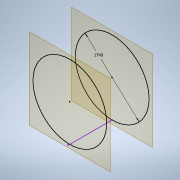
# Autodesk Inventor part: bok
Saved by Autodesk Inventor 2021 (Build 250183000, 183)
## iProperties
Created: 2021-09-19
Part Number: bok
Material: Ogólny
Document SubType Name: Konstrukcja blachowa
Designer: wojwo
Density: 1 g/cm^3
Sheet Metal Rule: Domyślny
Appearance: Domyślna
Author: wojwo
Autodesk Inventor part; units mm, degrees
ref_plane "XZ Plane" through (0, 0, 0) normal (0, 1, 0) x (-1, 0, 0)
sketch "Szkic1" plane through (0, 0, 0) normal (0, 0, 1) x (1, 0, 0)
  circle A0 centre (0, 0) radius 870
  line L0 (-870, 0) -> (870, 0) construction
  line L1 (0, -870) -> (0, 870) construction
  dimension "d0" = 1740
  constraints: 4 end point, 4 point on circle, 1 centre point, 1 coincident, 1 horizontal, 1 perpendicular
  measures "d0" diameter of A0
ref_plane "Płaszczyzna konstrukcyjna1" through (0, 0, 1000) normal (0, 0, 1) x (1, 0, 0)
sketch "Szkic2" plane through (0, 0, 1000) normal (0, 0, 1) x (1, 0, 0)
  circle A0 centre (0, 0) radius 870
  circle A1 centre (0, 0) radius 870
  line L0 (0, -870) -> (0, 870) construction
  line L1 (-870, 0) -> (870, 0) construction
  constraints: 4 end point, 4 point on circle, 2 centre point, 1 coincident
loft "Wyciągnięcie złożone1" add profiles "Szkic1", "Szkic2"
shell "Skorupa1" thickness 1 removed faces 2 at (213.0416, -16.8792, 1000) at (213.0416, -16.8792, 0)
equation "\"PromieńGięcia\" = Grubość"
equation "\"SzerokośćGięciaPodcięcia\" = Grubość"
equation "\"GłębokośćGięciaPodcięcia\" = 0.5 * Grubość"
equation "\"RozmiarPodcięciaNarożnika\" = 4 * Grubość"
equation "\"MinimalnaPozostałość\" = 2 * Grubość"
equation "\"PromieńPrzejścia\" = PromieńGięcia"
equation "\"Rozmiar_promienia_Jacobiego\" = Grubość"
equation "\"Wielk_odstępu\" = Grubość"
equation "\"Grubość\" = 0.5"
